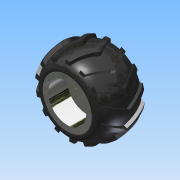
# Autodesk Inventor part: LargeRightWheel
Saved by Autodesk Inventor 2014 (Build 180170000, 170)
## iProperties
Created: 2011-09-20
Part Number: LargeRightWheel
Document SubType Name: Modeling
Designer: dgitz
Density: 1 g/cm^3
Material: Generic
Appearance: Default
Author: dgitz
Autodesk Inventor part; units mm, degrees
ref_plane "YZ Plane" through (0, 0, 0) normal (1, 0, 0) x (0, 1, 0)
sketch "Sketch1" plane through (0, 0, 0) normal (0, 0, 1) x (1, 0, 0)
  circle A0 centre (0, 0) radius 33.02
  circle A1 centre (0, 0) radius 36.068
  dimension "d0" = 66.04
  dimension "d1" = 72.136
  constraints: 2 centre point, 2 coincident
  measures "d0" diameter of A0
  measures "d1" diameter of A1
extrude "Extrusion1" add sketch "Sketch1" along normal blind 37.592
sketch "Sketch2" plane through (0, 0, 37.592) normal (0, 0, 1) x (1, 0, 0)
  circle A0 centre (0, 0) radius 36.068 projected
  circle A1 centre (0, 0) radius 36.068
  constraints: 1 centre point, 1 coincident, 1 concentric
extrude "Extrusion2" add sketch "Sketch2" along normal blind 8.2804
sketch "Sketch3" plane through (0, 0, 45.8724) normal (0, 0, 1) x (1, 0, 0)
  circle A0 centre (0, 0) radius 36.068 projected
  circle A1 centre (0, 0) radius 10.4648
  circle A2 centre (0, 0) radius 1.905
  dimension "d6" = 20.9296
  dimension "d7" = 3.81
  constraints: 2 centre point, 2 coincident
  measures "d6" diameter of A1
  measures "d7" diameter of A2
extrude "Extrusion3" add sketch "Sketch3" along normal blind 7.874 contours A1
sketch "Sketch4" plane through (0, 0, 45.8724) normal (0, 0, 1) x (1, 0, 0)
  circle A0 centre (0, 0) radius 36.068 projected
  circle A1 centre (0, 0) radius 10.4648 projected
  circle A2 centre (0, 0) radius 36.068
  circle A3 centre (0, 0) radius 33.02
  dimension "d10" = 66.04
  constraints: 2 centre point, 2 coincident, 1 concentric
  measures "d10" diameter of A3
extrude "Extrusion4" add sketch "Sketch4" along normal blind 33.3756 contours A0
sketch "Sketch5" plane through (0, 0, 37.592) normal (0, 0, -1) x (-1, 0, 0)
  circle A0 centre (0, 0) radius 33.02 projected
  line L0 (2.1997, -3.81) -> (-2.1997, -3.81)
  line L1 (-2.1997, -3.81) -> (-4.3994, 0)
  line L2 (-4.3994, 0) -> (-2.1997, 3.81)
  line L3 (-2.1997, 3.81) -> (2.1997, 3.81)
  line L4 (2.1997, 3.81) -> (4.3994, 0)
  line L5 (4.3994, 0) -> (2.1997, -3.81)
  dimension "d13" = 7.62
  constraints: 12 end point, 1 coincident, 1 horizontal, 13 other
  measures "d13" distance between parallel lines of L0 L3
extrude "Extrusion5" cut sketch "Sketch5" against normal blind 10.414 contours L0 L1 L2 L3 L4 L5
sketch "Sketch6" plane through (0, 0, 37.592) normal (0, 0, -1) x (-1, 0, 0)
  circle A0 centre (0, 0) radius 33.02 projected
  circle A1 centre (0, 0) radius 16.891
  circle A2 centre (0, 0) radius 33.02 projected
  line L0 (0.635, 33.0139) -> (0.635, 18.1499)
  line L1 (-0.635, 18.1499) -> (-0.635, 33.0139)
  line L2 (-28.9084, -15.957) -> (-16.0358, -8.525)
  line L3 (-15.4008, -9.6249) -> (-28.2734, -17.0569)
  line L4 (28.2734, -17.0569) -> (15.4008, -9.6249)
  line L5 (16.0358, -8.525) -> (28.9084, -15.957)
  arc A3 (-0.635, 18.1499) -> (-16.0358, -8.525) centre (0, 0) ccw
  arc A4 (-15.4008, -9.6249) -> (15.4008, -9.6249) centre (0, 0) ccw
  arc A5 (16.0358, -8.525) -> (0.635, 18.1499) centre (0, 0) ccw
  arc A6 (0.635, 33.0139) -> (-0.635, 33.0139) centre (0, 0) ccw
  arc A7 (-28.9084, -15.957) -> (-28.2734, -17.0569) centre (0, 0) ccw
  arc A8 (28.2734, -17.0569) -> (28.9084, -15.957) centre (0, 0) ccw
  dimension "d16" = 33.782
  dimension "d18" = 1.27
  dimension "d19" = 0.635
  dimension "d22" = 360
  constraints: 14 point on circle, 12 end point, 7 centre point, 3 coincident, 1 parallel, 1 vertical, 19 other
  measures "d16" diameter of A1
  measures "d18" distance between parallel lines of L0 L1
  measures "d19" distance from line of A0.centre L1
extrude "Extrusion6" add sketch "Sketch6" along normal blind 8.128 contours L0 A5 L5 A0 L4 A4 L3 L2 A3 L1
sketch "Sketch7" plane through (0, 0, 0) normal (1, 0, 0) x (0, 1, 0)
  line L0 (-10.4648, 45.8724) -> (-10.4648, 53.7464) projected
  line L1 (-10.4648, 53.7464) -> (-1.905, 53.7464) projected
  line L2 (-1.905, 53.7464) -> (-1.905, 48.006) projected
  line L3 (-1.905, 48.006) -> (-3.81, 48.006) projected
  line L4 (-3.81, 48.006) -> (-3.81, 37.592) projected
  line L5 (-3.81, 37.592) -> (-16.891, 37.592) projected
  line L6 (-16.891, 37.592) -> (-16.891, 29.464) projected
  line L7 (-16.891, 29.464) -> (-18.161, 29.464) projected
  line L8 (-18.161, 29.464) -> (-18.161, 37.592) projected
  line L9 (-18.161, 37.592) -> (-33.02, 37.592) projected
  line L10 (-33.02, 37.592) -> (-33.02, 0) projected
  line L11 (-33.02, 0) -> (-36.068, 0) projected
  line L12 (-36.068, 0) -> (-36.068, 79.248) projected
  line L13 (-36.068, 79.248) -> (-33.02, 79.248) projected
  line L14 (-33.02, 79.248) -> (-33.02, 45.8724) projected
  line L15 (-33.02, 45.8724) -> (-10.4648, 45.8724) projected
  line L16 (10.4648, 53.7464) -> (10.4648, 45.8724) projected
  line L17 (10.4648, 45.8724) -> (33.02, 45.8724) projected
  line L18 (33.02, 45.8724) -> (33.02, 79.248) projected
  line L19 (33.02, 79.248) -> (36.068, 79.248) projected
  line L20 (36.068, 79.248) -> (36.068, 0) projected
  line L21 (36.068, 0) -> (33.02, 0) projected
  line L22 (33.02, 0) -> (33.02, 29.464) projected
  line L23 (33.02, 29.464) -> (16.891, 29.464) projected
  line L24 (16.891, 29.464) -> (16.891, 37.592) projected
  line L25 (16.891, 37.592) -> (3.81, 37.592) projected
  line L26 (3.81, 37.592) -> (3.81, 48.006) projected
  line L27 (3.81, 48.006) -> (1.905, 48.006) projected
  line L28 (1.905, 48.006) -> (1.905, 53.7464) projected
  line L29 (1.905, 53.7464) -> (10.4648, 53.7464) projected
  line L30 (36.068, 79.248) -> (36.068, 0)
  line L31 (-36.068, 79.248) -> (36.068, 79.248) projected
  line L32 (-36.068, 0) -> (36.068, 0) projected
  line L33 (36.068, 79.248) -> (42.672, 79.248)
  line L34 (36.068, 0) -> (42.672, 0)
  line L35 (0, 98.0875) -> (0, -23.6959) construction
  line L36 (-10.4648, 45.8724) -> (-10.4648, 53.7464) construction
  line L37 (-10.4648, 53.7464) -> (-1.905, 53.7464) construction
  line L38 (-1.905, 53.7464) -> (-1.905, 48.006) construction
  line L39 (-1.905, 48.006) -> (-3.81, 48.006) construction
  line L40 (-3.81, 37.592) -> (-16.891, 37.592) construction
  line L41 (-16.891, 37.592) -> (-16.891, 29.464) construction
  line L42 (-16.891, 29.464) -> (-18.161, 29.464) construction
  line L43 (-18.161, 29.464) -> (-18.161, 37.592) construction
  line L44 (-18.161, 37.592) -> (-33.02, 37.592) construction
  line L45 (-33.02, 37.592) -> (-33.02, 0) construction
  line L46 (-33.02, 0) -> (-36.068, 0) construction
  line L47 (-36.068, 0) -> (-36.068, 79.248) construction
  line L48 (-36.068, 79.248) -> (-33.02, 79.248) construction
  line L49 (-33.02, 79.248) -> (-33.02, 45.8724) construction
  line L50 (-33.02, 45.8724) -> (-10.4648, 45.8724) construction
  line L51 (10.4648, 53.7464) -> (10.4648, 45.8724) construction
  line L52 (10.4648, 45.8724) -> (33.02, 45.8724) construction
  line L53 (33.02, 45.8724) -> (33.02, 79.248) construction
  line L54 (33.02, 79.248) -> (36.068, 79.248) construction
  line L55 (36.068, 79.248) -> (36.068, 0) construction
  line L56 (36.068, 0) -> (33.02, 0) construction
  line L57 (33.02, 0) -> (33.02, 29.464) construction
  line L58 (33.02, 29.464) -> (16.891, 29.464) construction
  line L59 (16.891, 29.464) -> (16.891, 37.592) construction
  line L60 (16.891, 37.592) -> (3.81, 37.592) construction
  line L61 (3.81, 48.006) -> (1.905, 48.006) construction
  line L62 (1.905, 48.006) -> (1.905, 53.7464) construction
  line L63 (1.905, 53.7464) -> (10.4648, 53.7464) construction
  line L64 (-10.4648, 45.8724) -> (-10.4648, 53.7464) construction
  line L65 (-10.4648, 53.7464) -> (-1.905, 53.7464) construction
  line L66 (-1.905, 53.7464) -> (-1.905, 48.006) construction
  line L67 (-1.905, 48.006) -> (-3.81, 48.006) construction
  line L68 (-3.81, 37.592) -> (-16.891, 37.592) construction
  line L69 (-16.891, 37.592) -> (-16.891, 29.464) construction
  line L70 (-16.891, 29.464) -> (-18.161, 29.464) construction
  line L71 (-18.161, 29.464) -> (-18.161, 37.592) construction
  line L72 (-18.161, 37.592) -> (-33.02, 37.592) construction
  line L73 (-33.02, 37.592) -> (-33.02, 0) construction
  line L74 (-33.02, 0) -> (-36.068, 0) construction
  line L75 (-36.068, 0) -> (-36.068, 79.248) construction
  line L76 (-36.068, 79.248) -> (-33.02, 79.248) construction
  line L77 (-33.02, 79.248) -> (-33.02, 45.8724) construction
  line L78 (-33.02, 45.8724) -> (-10.4648, 45.8724) construction
  line L79 (10.4648, 53.7464) -> (10.4648, 45.8724) construction
  line L80 (10.4648, 45.8724) -> (33.02, 45.8724) construction
  line L81 (33.02, 45.8724) -> (33.02, 79.248) construction
  line L82 (33.02, 79.248) -> (36.068, 79.248) construction
  line L83 (36.068, 79.248) -> (36.068, 0) construction
  line L84 (36.068, 0) -> (33.02, 0) construction
  line L85 (33.02, 0) -> (33.02, 29.464) construction
  line L86 (33.02, 29.464) -> (16.891, 29.464) construction
  line L87 (16.891, 29.464) -> (16.891, 37.592) construction
  line L88 (16.891, 37.592) -> (3.81, 37.592) construction
  line L89 (3.81, 48.006) -> (1.905, 48.006) construction
  line L90 (1.905, 48.006) -> (1.905, 53.7464) construction
  line L91 (1.905, 53.7464) -> (10.4648, 53.7464) construction
  line L92 (-36.068, 79.248) -> (-36.068, 0)
  line L93 (-36.068, 79.248) -> (-42.672, 79.248)
  line L94 (-36.068, 0) -> (-42.672, 0)
  ellipse E0 centre (45.4728, 39.624) end of major axis (27.4456, 39.624) minor radius 40.1111 (42.672, 0) -> (42.672, 79.248) ccw
  ellipse E1 centre (-45.4728, 39.624) end of major axis (-27.4456, 39.624) minor radius 40.1111 (-42.672, 79.248) -> (-42.672, 0) ccw
  line L95 (-63.5, 14.7973) -> (-63.5, 63.5963) construction
  line L96 (63.5, 9.0713) -> (63.5, 59.5395) construction
  line L97 (-3.81, 48.006) -> (-3.81, 37.592) projected
  line L98 (3.81, 37.592) -> (3.81, 48.006) projected
  line L99 (-3.81, 48.006) -> (-3.81, 37.592) projected
  line L100 (3.81, 37.592) -> (3.81, 48.006) projected
  point P0 (0, 0)
  dimension "d26" = 6.604
  dimension "d27" = 6.604
  dimension "d31" = 127
  constraints: 18 end point, 5 point on line, 5 symmetric about line, 5 vertical, 2 parallel, 1 horizontal, 1 perpendicular, 8 other
  measures "d26" distance of L30.start L33.end
  measures "d27" distance of L30.end L34.end
  measures "d31" distance between parallel lines of L96 L95
revolve "Revolution1" add sketch "Sketch7" angle 360 about axis through (0, 0, 98.0875) along (0, 0, -1) contours L12 L94 E1 L93 | L33 E0 L34 L20
sketch "Sketch8" plane through (0, 0, 45.8724) normal (0, 0, 1) x (1, 0, 0)
  circle A0 centre (0, 0) radius 33.02 projected
  circle A1 centre (0, 16.7005) radius 4.7625
  circle A2 centre (0, 0) radius 1.905 construction
  line L0 (0, 0) -> (0, 23.6357) construction
  circle A3 centre (-11.809, 11.809) radius 4.7625
  circle A4 centre (-16.7005, 0) radius 4.7625
  circle A5 centre (-11.809, -11.809) radius 4.7625
  circle A6 centre (0, -16.7005) radius 4.7625
  circle A7 centre (11.809, -11.809) radius 4.7625
  circle A8 centre (16.7005, 0) radius 4.7625
  circle A9 centre (11.809, 11.809) radius 4.7625
  dimension "d33" = 9.525
  dimension "d34" = 16.7005
  dimension "d37" = 360
  constraints: 8 centre point, 2 end point, 1 point on line, 1 vertical, 17 other
  measures "d33" diameter of A1
  measures "d34" distance of A0.centre A1.centre
extrude "Extrusion7" cut sketch "Sketch8" against normal blind 5.334 contours A1 | A3 | A4 | A5 | A6 | A7 | A8 | A9
ref_plane "Work Plane1" through (0, 68.58, 0) normal (0, 1, 0) x (-1, 0, 0)
ref_plane "Work Plane2" through (0, 0, 39.624) normal (0, 0, 1) x (1, 0, 0)
sketch "Sketch9" plane through (0, 68.58, 0) normal (0, 1, 0) x (-1, 0, 0)
  line L0 (0, 0) -> (-42.672, 0) construction
  line L1 (-5.334, 22.0746) -> (-5.334, 39.1465) construction
  line L2 (-15.748, 46.101) -> (-10.668, 46.101)
  line L3 (7.62, 4.191) -> (-0.508, 4.191)
  line L4 (-0.508, 4.191) -> (-18.288, 39.9583)
  line L5 (-18.288, 39.9583) -> (-15.748, 46.101)
  line L6 (-10.668, 46.101) -> (-10.668, 39.9583)
  line L7 (-10.668, 39.9583) -> (7.62, 4.191)
  line L8 (-18.288, 39.9583) -> (-10.668, 39.9583) construction
  point P0 (-14.478, 39.9583)
  dimension "d56" = 62.919
  dimension "d57" = 63.568
  dimension "d58" = 67.535
  dimension "d59" = 4.191
  dimension "d60" = 39.9583
  dimension "d61" = 46.101
  dimension "d62" = 5.334
  dimension "d63" = 8.6925
  dimension "d64" = 1.4107
  dimension "d65" = 39.1465
  dimension "d66" = 22.0746
  dimension "d67" = 39.9583
  dimension "d68" = 3.3923
  constraints: 16 end point, 4 parallel, 1 perpendicular
  measures "d56" angle of L7 L0
  measures "d57" angle of L4 L0
  measures "d58" angle of L5 L0
  measures "d59" distance between parallel lines of L3 L0
  measures "d60" distance between parallel lines of L8 L0
  measures "d61" distance between parallel lines of L2 L0
  measures "d62" distance between parallel lines of L6 L1
  measures "d63" distance from line of L0.start L7
  measures "d64" distance from line of L0.start L4
  measures "d65" distance from line of L1.end L0
  measures "d66" distance from line of L1.start L0
  measures "d67" distance from line of point (-14.478, 39.958) L0
  measures "d68" distance from line of point (-14.478, 39.958) L7
extrude "Extrusion8" add sketch "Sketch9" against normal up to next
mirror "Mirror3" about plane through (0, 0, 39.624) normal (0, 0, 1) of "Extrusion8"
pattern_circular "Circular Pattern2" count 14 over 360 about axis through (0, 0, 45.8724) along (0, 0, 1) of "Extrusion8", "Mirror3"
sketch "Sketch11" plane through (0, 0, 0) normal (1, 0, 0) x (0, 1, 0)
  line L0 (62.193, 54.6185) -> (65.532, 54.6185)
  line L1 (54.3517, 80.0428) -> (85.5873, 84.7088)
  line L2 (85.5873, 84.7088) -> (70.7723, 29.2632)
  spline S0 degree 2 poles (54.3517, 80.0428) (67.7292, 73.7281) (70.7723, 29.2632) knots 0 0 0 1 1 1
  line L3 (0, -16.9273) -> (0, 98.1545) projected
  point P0 (0, 0)
  point P1 (62.3954, 71.0588)
  dimension "d73" = 70.7723
  constraints: 6 end point, 3 other
  measures "d73" distance from line of L3 L2.end
revolve "Revolution3" cut sketch "Sketch11" angle 360 about axis through (0, 0, -10) along (0, 0, 1)
mirror "Mirror4" about plane through (0, 0, 39.624) normal (0, 0, 1) of "Revolution3"
body "Solid1"
